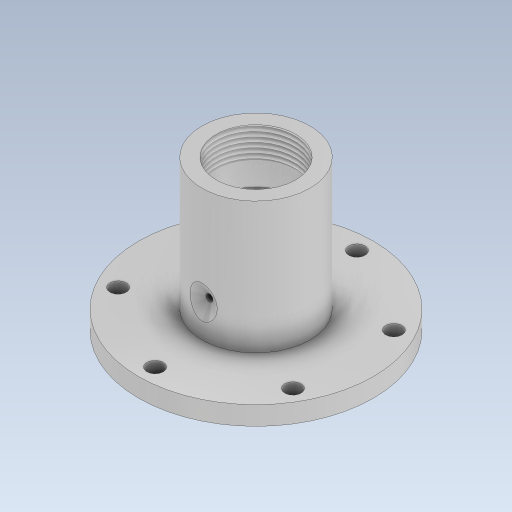
# Autodesk Inventor part: Pump-Motor-CW-Rotation:Casing 101
Saved by Autodesk Inventor 2024.2 (Build 282272000, 272)
## iProperties
Created: 2025-06-16
Material: Aluminum 6061
Document SubType Name: Modeling
Density: 2.7 g/cm^3
Appearance: Aluminum - Polished
Designer: cw
Author: cw
Autodesk Inventor part; units mm, degrees
note: some values were not read from the file. Chosen so that the rebuilt part matches the saved one: direction of "Hole3".
ref_plane "YZ Plane" through (0, 0, 0) normal (1, 0, 0) x (0, 1, 0)
ref_plane "XY Plane" through (0, 0, 0) normal (0, 0, 1) x (1, 0, 0)
sketch "Sketch1" plane through (0, 0, 0) normal (0, 1, 0) x (-1, 0, 0)
  line L0 (0, -36.5) -> (-23, -36.5)
  line L1 (-23, -36.5) -> (-23, 36.5)
  line L2 (-23, 36.5) -> (0, 36.5)
  line L3 (0, 36.5) -> (0, -36.5)
  line L4 (-23, -30.5) -> (-36, -30.5)
  line L5 (-36, -30.5) -> (-36, -27.5)
  line L6 (-36, -27.5) -> (-50, -27.5)
  line L7 (-50, -27.5) -> (-50, -19.5)
  line L8 (-50, -19.5) -> (-23, -19.5)
  point P0 (0, 0)
  point P1 (0, 0)
  dimension "d0" = 73
  dimension "d1" = 46
  dimension "d2" = 72
  dimension "d3" = 100
  dimension "d5" = 3
  dimension "d6" = 8
  dimension "d41" = 9
  constraints: 18 end point, 5 perpendicular, 2 horizontal, 2 parallel, 2 point on line, 1 coincident, 1 midpoint
  measures "d0" distance between parallel lines of L0 L2
  measures "d1" diameter of L1 L3
  measures "d2" diameter of L5 L3
  measures "d3" diameter of L7 L3
  measures "d5" distance between parallel lines of L6 L4
  measures "d6" distance between parallel lines of L8 L6
  measures "d41" vertical distance of L6.end L0.end
revolve "Revolution1" add sketch "Sketch1" angle 360 about axis through (0, 0, 36.5) along (0, 0, -1)
sketch "Sketch2" plane through (0, 0, -36.5) normal (0, 0, -1) x (-1, 0, 0)
  point P0 (0, 0)
hole "Hole1" at (0, 0, -36.5) direction (0, 0, 1) diameter 25 end through all
sketch "Sketch3" plane through (0, 0, 36.5) normal (0, 0, 1) x (1, 0, 0)
  point P0 (0, 0)
hole "Hole2" at (0, 0, 36.5) direction (0, 0, -1) diameter 33.835 depth 23 thread size "M36x2" class "6H" standard "ISO Metric profile"
ref_plane "Work Plane1" through (0, -23, 8.5) normal (0, 1, 0) x (-1, 0, 0)
sketch "Sketch4" plane through (0, -23, 8.5) normal (0, 1, 0) x (-1, 0, 0)
  line L0 (23, 28) -> (-23, 28) construction
  point P0 (0, -8.5)
  point P1 (0, -14)
  dimension "d22" = 42
  constraints: 1 vertical alignment
  measures "d22" distance from line of point (0, -14) L0
hole "Hole3" at (0, -23, -5.5) direction (0, 1, 0) diameter 3 end up to surface countersink diameter 14 countersink angle 120
sketch "Sketch5" plane through (0, 0, -19.5) normal (0, 0, 1) x (1, 0, 0)
  circle A0 centre (0, 0) radius 12.5 projected
  circle A1 centre (0, 0) radius 43 construction
  point P0 (0, 0)
  point P1 (0, -43)
  dimension "d30" = 86
  constraints: 2 vertical alignment, 1 coincident, 2 other
hole "Hole4" at (0, -43, -19.5) direction (0, 0, -1) diameter 7 end through all
pattern_circular "Circular Pattern1" count 6 over 360 about axis through (0, 0, -10) along (0, 0, 1) of "Hole4"
body "Solid1"
